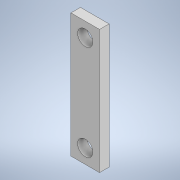
# Autodesk Inventor part: リンク26×6×2
Saved by Autodesk Inventor 2021 (Build 250183000, 183)
## iProperties
Created: 2021-10-09
Part Number: リンク26×6×2
Material: 一般
Document SubType Name: Modeling
Designer: ryusei
Density: 1 g/cm^3
Appearance: 既定
Author: ryusei
Autodesk Inventor part; units mm, degrees
ref_plane "YZ Plane" through (0, 0, 0) normal (1, 0, 0) x (0, 1, 0)
ref_plane "XZ Plane" through (0, 0, 0) normal (0, 1, 0) x (-1, 0, 0)
ref_plane "XY Plane" through (0, 0, 0) normal (0, 0, 1) x (1, 0, 0)
sketch "スケッチ1" plane through (0, 0, 0) normal (0, 0, 1) x (1, 0, 0)
  line L0 (0, 0) -> (6, 0)
  line L1 (6, 0) -> (6, 30)
  line L2 (6, 30) -> (0, 30)
  line L3 (0, 30) -> (0, 0)
  dimension "d0" = 6
  dimension "d1" = 30
  constraints: 8 end point, 2 parallel, 1 horizontal, 1 perpendicular
  measures "d0" distance of L0.start L0.end
  measures "d1" distance of L0.end L1.end
extrude "押し出し1" add sketch "スケッチ1" along normal blind 2
sketch "スケッチ2" plane through (0, 0, 2) normal (0, 0, 1) x (1, 0, 0)
  line L0 (6, 30) -> (0, 30) projected
  line L1 (6, 0) -> (6, 30) projected
  line L2 (0, 0) -> (6, 0) projected
  point P0 (3, 25)
  point P1 (3, 5)
  dimension "d4" = 5
  dimension "d5" = 3
  dimension "d6" = 3
  dimension "d7" = 5
  measures "d4" distance from line of L0 point (3, 25)
  measures "d5" distance from line of L1 point (3, 25)
  measures "d6" distance from line of L1 point (3, 5)
  measures "d7" distance from line of L2 point (3, 5)
hole "穴1" at (3, 25, 2) at (3, 5, 2) direction (0, 0, -1) diameter 3.2 end through all
sketch "スケッチ4" plane through (0, 0, 2) normal (0, 0, 1) x (1, 0, 0)
  line L0 (6, 30) -> (0, 30) projected
  line L1 (6, 0) -> (6, 30) projected
  line L2 (0, 30) -> (6, 30)
  line L3 (6, 30) -> (6, 28)
  line L4 (6, 28) -> (0, 28)
  line L5 (0, 28) -> (0, 30)
  line L6 (0, 30) -> (0, 0) projected
  line L7 (0, 2) -> (6, 2)
  line L8 (6, 2) -> (6, 0)
  line L9 (6, 0) -> (0, 0)
  line L10 (0, 0) -> (0, 2)
  dimension "d18" = 2
  dimension "d19" = 2
  constraints: 16 end point, 4 parallel, 2 horizontal, 2 perpendicular, 2 point on line
  measures "d18" distance between parallel lines of L0 L4
  measures "d19" distance between parallel lines of L9 L7
extrude "押し出し2" cut sketch "スケッチ4" against normal blind 10 contours L1 L4 L5 L0 | L1 L9 L6 L7
